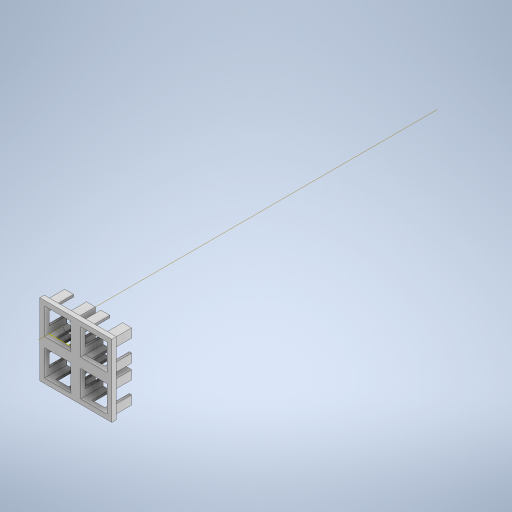
# Autodesk Inventor part: retainer test
Saved by Autodesk Inventor 2024 (Build 280153000, 153)
## iProperties
Created: 2024-03-20
Part Number: retainer test
Material: Generic
Document SubType Name: Modeling
Designer: drew
Density: 1 g/cm^3
Appearance: Default
Author: drew
Autodesk Inventor part; units mm, degrees
ref_plane "YZ Plane" through (0, 0, 0) normal (1, 0, 0) x (0, 1, 0)
ref_plane "XZ Plane" through (0, 0, 0) normal (0, 1, 0) x (-1, 0, 0)
ref_plane "XY Plane" through (0, 0, 0) normal (0, 0, 1) x (1, 0, 0)
sketch "Sketch1" plane through (0, 0, 0) normal (0, 1, 0) x (-1, 0, 0)
  line L0 (-1.009, 1.009) -> (1.009, 1.009)
  line L1 (1.009, 1.009) -> (1.009, -1.009)
  line L2 (1.009, -1.009) -> (-1.009, -1.009)
  line L3 (-1.009, -1.009) -> (-1.009, 1.009)
  line L4 (-1.009, 1.009) -> (1.009, -1.009) construction
  line L5 (1.009, 1.009) -> (-1.009, -1.009) construction
  line L6 (0.9364, 0.9364) -> (0.0764, 0.9364)
  line L7 (0.0764, 0.9364) -> (0.0764, 0.0764)
  line L8 (0.0764, 0.0764) -> (0.9364, 0.0764)
  line L9 (0.9364, 0.0764) -> (0.9364, 0.9364)
  line L10 (0, 0) -> (0.3282, 0)
  line L11 (0.8739, 0.8739) -> (0.1389, 0.8739)
  line L12 (0.1389, 0.8739) -> (0.1389, 0.1389)
  line L13 (0.1389, 0.1389) -> (0.8739, 0.1389)
  line L14 (0.8739, 0.1389) -> (0.8739, 0.8739)
  line L15 (-1.009, 1.009) -> (1.009, -1.009) construction
  line L16 (-0.0764, 0.9364) -> (-0.9364, 0.9364)
  line L17 (-0.1389, 0.8739) -> (-0.8739, 0.8739)
  line L18 (-0.8739, 0.8739) -> (-0.8739, 0.1389)
  line L19 (-0.8739, 0.1389) -> (-0.1389, 0.1389)
  line L20 (-0.9364, 0.9364) -> (-0.9364, 0.0764)
  line L21 (-0.9364, 0.0764) -> (-0.0764, 0.0764)
  line L22 (-0.0764, 0.0764) -> (-0.0764, 0.9364)
  line L23 (-0.1389, 0.1389) -> (-0.1389, 0.8739)
  line L24 (-1.009, -1.009) -> (1.009, 1.009) construction
  line L25 (-0.9364, -0.0764) -> (-0.9364, -0.9364)
  line L26 (-0.8739, -0.1389) -> (-0.8739, -0.8739)
  line L27 (-0.8739, -0.8739) -> (-0.1389, -0.8739)
  line L28 (-0.1389, -0.8739) -> (-0.1389, -0.1389)
  line L29 (-0.9364, -0.9364) -> (-0.0764, -0.9364)
  line L30 (-0.0764, -0.9364) -> (-0.0764, -0.0764)
  line L31 (-0.0764, -0.0764) -> (-0.9364, -0.0764)
  line L32 (-0.1389, -0.1389) -> (-0.8739, -0.1389)
  line L33 (1.009, -1.009) -> (-1.009, 1.009) construction
  line L34 (0.0764, -0.9364) -> (0.9364, -0.9364)
  line L35 (0.1389, -0.8739) -> (0.8739, -0.8739)
  line L36 (0.8739, -0.8739) -> (0.8739, -0.1389)
  line L37 (0.8739, -0.1389) -> (0.1389, -0.1389)
  line L38 (0.9364, -0.9364) -> (0.9364, -0.0764)
  line L39 (0.9364, -0.0764) -> (0.0764, -0.0764)
  line L40 (0.0764, -0.0764) -> (0.0764, -0.9364)
  line L41 (0.1389, -0.1389) -> (0.1389, -0.8739)
  dimension "d0" = 2.018
  dimension "d2" = 0.1529
  dimension "d3" = 0.86
  dimension "d4" = 0.0625
  dimension "d7" = 360
  constraints: 84 end point, 8 point on line, 6 parallel, 4 perpendicular, 3 horizontal, 2 coincident, 2 midpoint, 82 other
  measures "d0" distance of L0.end L1.end
  measures "d2" diameter of L8 L10
  measures "d3" distance between parallel lines of L7 L9
  measures "d4" distance between parallel lines of L9 L14
extrude "Extrusion1" add sketch "Sketch1" along normal blind 0.125 contours L0 L1 L2 L3 | L9 L8 L7 L6 | L22 L21 L20 L16 | L31 L30 L29 L25 | L40 L39 L38 L34
sketch "Sketch2" plane through (0, 0.125, 0) normal (0, 1, 0) x (1, 0, 0)
  line L0 (1.009, 1.009) -> (-1.009, 1.009) projected
  line L1 (-1.009, 1.009) -> (-1.009, -1.009) projected
  line L2 (-1.009, -1.009) -> (1.009, -1.009) projected
  line L3 (1.009, -1.009) -> (1.009, 1.009) projected
  line L4 (-0.8739, -0.8739) -> (-0.8739, -0.1389) projected
  line L5 (-0.8739, -0.1389) -> (-0.1389, -0.1389) projected
  line L6 (-0.1389, -0.1389) -> (-0.1389, -0.8739) projected
  line L7 (-0.1389, -0.8739) -> (-0.8739, -0.8739) projected
  line L8 (0.1389, -0.8739) -> (0.1389, -0.1389) projected
  line L9 (0.1389, -0.1389) -> (0.8739, -0.1389) projected
  line L10 (0.8739, -0.1389) -> (0.8739, -0.8739) projected
  line L11 (0.8739, -0.8739) -> (0.1389, -0.8739) projected
  line L12 (0.8739, 0.1389) -> (0.1389, 0.1389) projected
  line L13 (0.1389, 0.1389) -> (0.1389, 0.8739) projected
  line L14 (0.1389, 0.8739) -> (0.8739, 0.8739) projected
  line L15 (0.8739, 0.8739) -> (0.8739, 0.1389) projected
  line L16 (-0.1389, 0.8739) -> (-0.1389, 0.1389) projected
  line L17 (-0.1389, 0.1389) -> (-0.8739, 0.1389) projected
  line L18 (-0.8739, 0.1389) -> (-0.8739, 0.8739) projected
  line L19 (-0.8739, 0.8739) -> (-0.1389, 0.8739) projected
  line L20 (-0.9364, -0.0764) -> (-0.9364, -0.9364)
  line L21 (-0.9364, -0.9364) -> (-0.0764, -0.9364)
  line L22 (-0.0764, -0.9364) -> (-0.0764, -0.0764)
  line L23 (-0.0764, -0.0764) -> (-0.9364, -0.0764)
  line L24 (-0.9364, -0.6864) -> (-0.8739, -0.6864)
  line L25 (-0.6864, -0.9364) -> (-0.6864, -0.8739)
  point P0 (0, 0)
  point P1 (-0.9052, -0.6864)
  dimension "d11" = 0.0625
  dimension "d12" = 0.25
  dimension "d13" = 0.25
  constraints: 12 end point, 4 point on line, 2 perpendicular, 1 midpoint, 3 other
  measures "d11" distance between parallel lines of L4 L20
  measures "d12" distance between parallel lines of L20 L25
  measures "d13" distance from line of L21 point (-0.905, -0.686)
extrude "Extrusion2" add sketch "Sketch2" along normal blind 0.5 contours L7 L25 L21 L20 L24 L4
sketch "Sketch3" plane through (0, 0.125, 0) normal (0, 1, 0) x (1, 0, 0)
  line L0 (-0.1389, -0.1389) -> (-0.1389, -0.8739) projected
  line L1 (-0.8739, -0.1389) -> (-0.1389, -0.1389) projected
  line L2 (-0.1389, -0.8739) -> (-0.8739, -0.1389) construction
  line L3 (-0.5064, -0.5064) -> (-0.1389, -0.1389) construction
  point P0 (0, 0)
  constraints: 4 end point, 1 midpoint
pattern_circular "Circular Pattern1" count 4 over 360 about axis through (-0.5064, 0.125, 0.5064) along (0, 1, 0) of "Extrusion2"
pattern_circular "Circular Pattern2" count 4 over 360 about axis through (0, -10, 0) along (0, 1, 0) of "Extrusion2", "Circular Pattern1"
body "Solid1"
